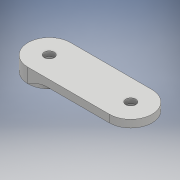
# Autodesk Inventor part: Arm - left actuator hinge
Saved by Autodesk Inventor 2017 (Build 210142000, 142)
## iProperties
Created: 2016-03-31
Part Number: Arm - left actuator hinge
Material: Generic
Document SubType Name: Modeling
Designer: alist
Density: 1 g/cm^3
Appearance: Default
Author: alist
Autodesk Inventor part; units mm, degrees
ref_plane "YZ Plane" through (0, 0, 0) normal (1, 0, 0) x (0, 1, 0)
ref_plane "XZ Plane" through (0, 0, 0) normal (0, 1, 0) x (-1, 0, 0)
ref_plane "XY Plane" through (0, 0, 0) normal (0, 0, 1) x (1, 0, 0)
sketch "Sketch1" plane through (0, 0, 0) normal (0, 0, 1) x (1, 0, 0)
  line L0 (-32.5, 0) -> (32.5, 0) construction
  line L1 (-32.5, -17) -> (32.5, -17)
  line L2 (32.5, 17) -> (-32.5, 17)
  arc A0 (-32.5, 17) -> (-32.5, -17) centre (-32.5, 0) ccw
  arc A1 (32.5, -17) -> (32.5, 17) centre (32.5, 0) ccw
  point P0 (0, 0)
  point P1 (0, 0)
  dimension "d0" = 65
  dimension "d1" = 34
  constraints: 8 end point, 4 point on circle, 4 tangent, 2 centre point, 1 coincident, 1 horizontal, 1 midpoint, 1 parallel
  measures "d0" distance of L0.start L0.end
  measures "d1" diameter of A1
extrude "Extrusion1" add sketch "Sketch1" along normal blind 6
sketch "Sketch2" plane through (0, 0, 0) normal (0, 0, -1) x (-1, 0, 0)
  arc A0 (32.5, -17) -> (32.5, 17) centre (32.5, 0) ccw projected
  circle A1 centre (32.5, 0) radius 17
  point P0 (0, 0)
  dimension "d4" = 34
  constraints: 1 centre point, 1 coincident
  measures "d4" diameter of A1
extrude "Extrusion2" add sketch "Sketch2" along normal blind 5.5
sketch "Sketch3" plane through (0, 0, 0) normal (0, 0, -1) x (-1, 0, 0)
  arc A0 (-32.5, 17) -> (-32.5, -17) centre (-32.5, 0) ccw projected
  circle A1 centre (-32.5, 0) radius 5.5
  point P0 (0, 0)
  dimension "d8" = 11
  constraints: 1 centre point, 1 coincident
  measures "d8" diameter of A1
extrude "Extrusion3" add sketch "Sketch3" along normal blind 1
sketch "Sketch4" plane through (32.5, 0, -1) normal (0, 0, -1) x (-1, 0, 0)
  circle A0 centre (0, 0) radius 4
  point P0 (32.5, 0)
  dimension "d11" = 8
  constraints: 1 centre point
  measures "d11" diameter of A0
extrude "Extrusion4" add sketch "Sketch4" along normal blind 3.5
chamfer "Chamfer1" distance 1 angle 45 1 edges at (36.5, 0, -4.5)
hole "Hole1" at (32.5, 0, 6) direction (0, 0, -1) diameter 4.3 end through all counterbore diameter 8 counterbore depth 4
chamfer "Chamfer2" distance 1.85 angle 45 1 edges at (32.5, 2.15, 2)
sketch "Sketch5" plane through (-32.5, 0, -5.5) normal (0, 0, -1) x (-1, 0, 0)
  circle A0 centre (0, 0) radius 5.5
  point P0 (-32.5, 0)
  dimension "d29" = 11
  constraints: 1 centre point
  measures "d29" diameter of A0
extrude "Extrusion5" add sketch "Sketch5" along normal blind 1
sketch "Sketch6" plane through (-32.5, 0, -6.5) normal (0, 0, -1) x (-1, 0, 0)
  circle A0 centre (0, 0) radius 4
  point P0 (-32.5, 0)
  dimension "d32" = 8
  constraints: 1 centre point
  measures "d32" diameter of A0
extrude "Extrusion6" add sketch "Sketch6" along normal blind 3.5
chamfer "Chamfer3" distance 1 angle 45 1 edges at (-28.5, 0, -10)
hole "Hole2" at (-32.5, 0, 6) direction (0, 0, -1) diameter 4.3 end through all counterbore diameter 8 counterbore depth 4
chamfer "Chamfer4" distance 1.85 angle 45 1 edges at (-32.5, 2.15, 2)
fillet "Fillet2" radius 5.5 1 edges at (-15.5, 0, 0)
body "Solid1"
